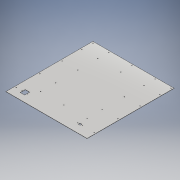
# Autodesk Inventor part: Back Cladding
Saved by Autodesk Inventor 2019 (Build 230136000, 136)
## iProperties
Created: 2018-10-13
Part Number: Back Cladding
Material: Aluminium 1050
Document SubType Name: Sheet Metal
Designer: Ax
Density: 2.7 g/cm^3
Sheet Metal Rule: Default_mm
Appearance: Aluminum - Dark
Mass: 1137.09 g
Surface Area: 5654.85 cm^2
Volume: 421.144 cm^3
Flat Pattern Width: 51.3 cm
Flat Pattern Length: 55 cm
Flat Pattern Area: 2821.5 cm^2
Sheet Metal Width: 513.000 mm
Sheet Metal Length: 550.000 mm
Sheet Metal Area: 282150.000 mm^2
Project: AX-01 CoreXY
Author: Ax
Autodesk Inventor part; units mm, degrees
ref_plane "YZ Plane" through (0, 0, 0) normal (1, 0, 0) x (0, 1, 0)
ref_plane "XZ Plane" through (0, 0, 0) normal (0, 1, 0) x (-1, 0, 0)
ref_plane "XY Plane" through (0, 0, 0) normal (0, 0, 1) x (1, 0, 0)
sketch "Sketch1" plane through (0, 0, 0) normal (0, 0, 1) x (1, 0, 0)
  line L0 (-256.5, -275) -> (256.5, -275)
  line L1 (256.5, -275) -> (256.5, 275)
  line L2 (256.5, 275) -> (-256.5, 275)
  line L3 (-256.5, 275) -> (-256.5, -275)
  line L4 (-256.5, -275) -> (256.5, 275) construction
  line L5 (256.5, -275) -> (-256.5, 275) construction
  line L6 (-256.5, 265) -> (256.5, 265) construction
  line L7 (-246.5, 275) -> (-246.5, -275) construction
  line L8 (246.5, 275) -> (246.5, -275) construction
  line L9 (-256.5, -165) -> (256.5, -165) construction
  line L10 (-256.5, 195) -> (256.5, 195) construction
  circle A0 centre (-246.5, 265) radius 2.1
  circle A1 centre (-146.5, 265) radius 2.1
  circle A2 centre (146.5, 265) radius 2.1
  circle A3 centre (246.5, 265) radius 2.1
  circle A4 centre (146.5, 195) radius 2.1
  circle A5 centre (246.5, 195) radius 2.1
  circle A6 centre (-246.5, 195) radius 2.1
  circle A7 centre (-146.5, 195) radius 2.1
  line L11 (-146.5, 275) -> (-146.5, -275) construction
  line L12 (0, 0) -> (0, -275) construction
  line L13 (146.5, 275) -> (146.5, -275) construction
  circle A8 centre (-246.5, 70) radius 2.1
  circle A9 centre (146.5, -165) radius 2.1
  circle A10 centre (-146.5, -165) radius 2.1
  circle A11 centre (-246.5, -70) radius 2.1
  circle A12 centre (-246.5, -220) radius 2.1
  circle A13 centre (246.5, -220) radius 2.1
  circle A14 centre (246.5, -70) radius 2.1
  circle A15 centre (246.5, 70) radius 2.1
  line L14 (-246.5, 70) -> (246.5, 70) construction
  line L15 (-246.5, -70) -> (246.5, -70) construction
  line L16 (-246.5, 0) -> (246.5, 0) construction
  line L17 (-246.5, -220) -> (246.5, -220) construction
  line L18 (0, 275) -> (0, 0) construction
  circle A16 centre (0, 265) radius 2.1
  circle A17 centre (0, 195) radius 2.1
  circle A18 centre (0, -165) radius 2.1
  circle A19 centre (-146.5, 70) radius 2.1
  circle A20 centre (146.5, 70) radius 2.1
  circle A21 centre (146.5, -70) radius 2.1
  circle A22 centre (-146.5, -70) radius 2.1
  dimension "d0" = 513
  dimension "d1" = 550
  dimension "d2" = 10
  dimension "d3" = 10
  dimension "d4" = 10
  dimension "d5" = 110
  dimension "d6" = 80
  dimension "d7" = 110
  dimension "d8" = 110
  dimension "d9" = 70
  dimension "d10" = 55
  dimension "d11" = 4.2
  measures "d0" distance of L1.end L2.end
  measures "d1" distance of L0.end L1.end
  measures "d2" distance of L2.end L6.start
  measures "d3" distance of L0.start L7.end
  measures "d4" distance of L0.end L8.end
  measures "d5" distance of L0.end L9.end
  measures "d6" distance of L10.end L1.end
  measures "d7" distance of L0.start L11.end
  measures "d8" distance of L13.end L0.end
  measures "d9" vertical distance of L12.start L14.start
  measures "d10" vertical distance of L0.end L17.end
  measures "d11" diameter of A7
extrude "Plate5" add sketch "Sketch1" along normal blind 1.5
sketch "Sketch2" plane through (0, 0, 1.5) normal (0, 0, 1) x (1, 0, 0)
  line L0 (-206.5, -203) -> (-178.5, -203)
  line L1 (-178.5, -203) -> (-178.5, -235)
  line L2 (-178.5, -235) -> (-206.5, -235)
  line L3 (-206.5, -235) -> (-206.5, -203)
  line L4 (-210.5, -219) -> (-174.5, -219) construction
  line L5 (-192.5, -203) -> (-192.5, -235) construction
  circle A0 centre (-210.5, -219) radius 1.7
  circle A1 centre (-174.5, -219) radius 1.7
  line L6 (-256.5, -275) -> (-256.5, 275) projected
  line L7 (256.5, -275) -> (-256.5, -275) projected
  point P0 (0, 0)
  point P1 (-178.5, -219)
  dimension "d22" = 32
  dimension "d23" = 28
  dimension "d24" = 36
  dimension "d25" = 3.4
  dimension "d26" = 50
  dimension "d30" = 56
  constraints: 12 end point, 3 midpoint, 2 centre point, 2 coincident, 2 horizontal, 2 parallel, 1 equal radius, 1 perpendicular, 1 point on line, 1 symmetric about line
  measures "d22" distance of L0.end L1.end
  measures "d23" distance of L0.start L0.end
  measures "d24" distance of L4.start L4.end
  measures "d25" diameter of A1
  measures "d26" distance between parallel lines of L3 L6
  measures "d30" distance between parallel lines of L7 L4
extrude "Cut1" cut sketch "Sketch2" against normal blind 1.5
sketch "Sketch3" plane through (0, 0, 1.5) normal (0, 0, 1) x (1, 0, 0)
  line L0 (141.5, -219) -> (171.5, -219) construction
  line L1 (256.5, -275) -> (-256.5, -275) projected
  line L2 (150.5, -224.625) -> (162.5, -224.625)
  line L3 (162.5, -224.625) -> (162.5, -213.375)
  line L4 (162.5, -213.375) -> (150.5, -213.375)
  line L5 (150.5, -213.375) -> (150.5, -224.625)
  line L6 (150.5, -224.625) -> (162.5, -213.375) construction
  line L7 (162.5, -224.625) -> (150.5, -213.375) construction
  circle A0 centre (141.5, -219) radius 1.75
  circle A1 centre (171.5, -219) radius 1.75
  line L8 (256.5, 275) -> (256.5, -275) projected
  point P0 (0, 0)
  point P1 (156.5, -219)
  dimension "d31" = 56
  dimension "d32" = 30
  dimension "d33" = 11.25
  dimension "d34" = 12
  dimension "d35" = 3.5
  dimension "d36" = 100
  constraints: 14 end point, 3 midpoint, 2 centre point, 2 coincident, 2 horizontal, 2 parallel, 1 equal radius, 1 perpendicular
  measures "d31" distance between parallel lines of L1 L0
  measures "d32" distance of L0.start L0.end
  measures "d33" distance of L2.end L3.end
  measures "d34" distance of L2.start L2.end
  measures "d35" diameter of A0
  measures "d36" distance from line of L8 point (156.5, -219)
extrude "Cut2" cut sketch "Sketch3" against normal blind 1.5
equation "\"d28\" = Thickness"
equation "\"d37\" = Thickness"
equation "\"d21\" = Thickness"
equation "\"CornerReliefSize\" = 4 * Thickness"
equation "\"TransitionRadius\" = BendRadius"
equation "\"JacobiRadiusSize\" = BendRadius"
equation "\"d12\" = BendRadius"
equation "\"d13\" = BendRadius"
equation "\"d16\" = BendRadius"
equation "\"d19\" = BendRadius"
equation "\"d20\" = BendRadius"
equation "\"Thickness\" = 1.5"
equation "\"BendRadius\" = 0.8"
body "Solid5"
